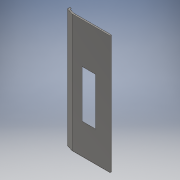
# Autodesk Inventor part: Cover Lower Front
Saved by Autodesk Inventor 2018 (Build 220112000, 112)
## iProperties
Created: 2018-08-07
Part Number: Cover Lower Front
Material: Steel
Document SubType Name: Modeling
Designer: P301319
Density: 7.85 g/cm^3
Appearance: Stainless - Brushed
Author: P301319
Autodesk Inventor part; units mm, degrees
ref_plane "YZ Plane" through (0, 0, 0) normal (1, 0, 0) x (0, 1, 0)
ref_plane "XZ Plane" through (0, 0, 0) normal (0, 1, 0) x (-1, 0, 0)
ref_plane "XY Plane" through (0, 0, 0) normal (0, 0, 1) x (1, 0, 0)
sketch "Sketch1" plane through (0, 0, 0) normal (0, 0, 1) x (1, 0, 0)
  line L0 (0, 0) -> (560, 0)
  line L1 (0, 0) -> (-100, 30)
  line L2 (0, 0) -> (104.4031, 0) construction
  line L3 (-100, 30) -> (-100, 67)
  line L4 (-98.4, 67) -> (-98.4, 31.1904)
  line L5 (-98.4, 31.1904) -> (0.2348, 1.6)
  line L6 (0.2348, 1.6) -> (560, 1.6)
  line L7 (-98.4, 67) -> (-100, 67)
  line L8 (560, 1.6) -> (560, 0)
  dimension "d0" = 560
  dimension "d2" = 100
  dimension "d3" = 37
  dimension "d9" = 30
  dimension "d10" = 1.6
  constraints: 18 end point, 3 horizontal, 2 vertical, 1 equal length, 2 other
  measures "d0" distance of L0.start L0.end
  measures "d2" horizontal distance of L0.start L1.end
  measures "d3" distance of L1.end L3.end
  measures "d9" vertical distance of L0.start L1.end
  measures "d10" distance between parallel lines of L1 L5
extrude "Extrusion1" add sketch "Sketch1" along normal blind 1750
sketch "Sketch2" plane through (0, 0, 1750) normal (0, 0, 1) x (1, 0, 0)
  line L0 (-98.4, 31.1904) -> (-98.4, 67) projected
  line L1 (0.2348, 1.6) -> (-98.4, 31.1904) projected
  line L2 (560, 1.6) -> (0.2348, 1.6) projected
  line L3 (-78.4, 67) -> (-78.4, 46.0711)
  line L4 (-78.4, 46.0711) -> (3.1702, 21.6)
  line L5 (3.1702, 21.6) -> (560, 21.6)
  line L6 (-78.4, 67) -> (-98.4, 67)
  line L7 (560, 21.6) -> (560, 1.6)
  line L8 (560, 1.6) -> (558.4, 1.6)
  line L9 (558.4, 1.6) -> (558.4, 21.6)
  line L10 (558.4, 21.6) -> (560, 21.6)
  line L11 (560, 21.6) -> (560, 1.6)
  point P0 (0, 0)
  dimension "d11" = 20
  dimension "d16" = 1.6
  dimension "d17" = 20
  constraints: 18 end point, 2 horizontal, 2 parallel, 1 perpendicular, 1 vertical, 2 other
  measures "d11" distance between parallel lines of L1 L4
  measures "d16" distance of L9.end L10.end
  measures "d17" distance of L8.end L9.end
extrude "Extrusion2" add sketch "Sketch2" against normal blind 1.6
sketch "Sketch3" plane through (0, 0, 0) normal (0, 0, -1) x (-1, 0, 0)
  line L0 (98.4, 67) -> (98.4, 31.1904) projected
  line L1 (98.4, 67) -> (78.4, 67) projected
  line L2 (78.4, 67) -> (78.4, 46.0711) projected
  line L3 (78.4, 46.0711) -> (-3.1702, 21.6) projected
  line L4 (-3.1702, 21.6) -> (-560, 21.6) projected
  line L5 (-560, 21.6) -> (-560, 1.6) projected
  line L6 (-0.2348, 1.6) -> (-560, 1.6) projected
  line L7 (98.4, 31.1904) -> (-0.2348, 1.6) projected
  point P0 (0, 0)
extrude "Extrusion3" add sketch "Sketch3" against normal blind 1.6
sketch "Sketch4" plane through (0, 0, 1748.4) normal (0, 0, -1) x (-1, 0, 0)
  line L0 (-560, 21.6) -> (-560, 1.6) projected
  line L1 (-560, 21.6) -> (-558.4, 21.6)
  line L2 (-558.4, 21.6) -> (-558.4, 1.6)
  line L3 (-558.4, 1.6) -> (-560, 1.6)
  line L4 (-560, 1.6) -> (-560, 21.6)
  point P0 (0, 0)
  dimension "d18" = 1.6
  dimension "d19" = 20
  constraints: 8 end point, 2 parallel, 1 horizontal, 1 perpendicular
  measures "d18" distance of L2.end L3.end
  measures "d19" distance of L1.end L2.end
extrude "Extrusion4" add sketch "Sketch4" along normal up to surface (1748.4 mm away)
sketch "Sketch5" plane through (0, 0, 0) normal (0, -1, 0) x (1, 0, 0)
  line L0 (146.0887, 450) -> (346.0887, 450)
  line L1 (346.0887, 450) -> (346.0887, 1150)
  line L2 (346.0887, 1150) -> (146.0887, 1150)
  line L3 (146.0887, 1150) -> (146.0887, 450)
  line L4 (0, 0) -> (560, 0) projected
  dimension "d22" = 200
  dimension "d23" = 700
  dimension "d24" = 450
  constraints: 8 end point, 2 parallel, 1 horizontal, 1 perpendicular
  measures "d22" distance of L2.end L1.end
  measures "d23" distance of L1.end L0.end
  measures "d24" distance between parallel lines of L0 L4
extrude "Extrusion5" cut sketch "Sketch5" against normal blind 10
body "Solid1"
